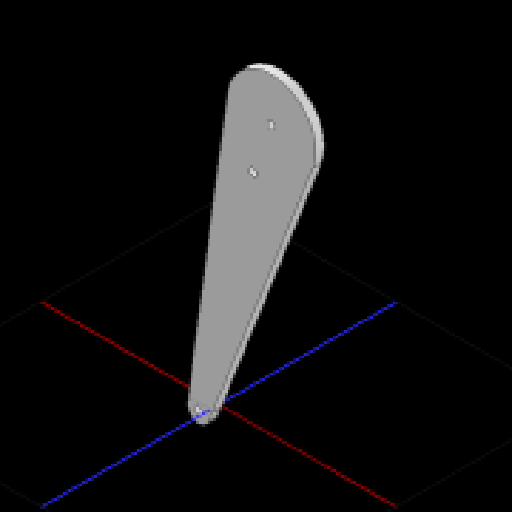
# Autodesk Inventor part: matchloaderbar
Saved by Autodesk Inventor 2025.2 (Build 292293000, 293)
## iProperties
Created: 2026-01-23
Part Number: matchloaderbar
Material: Generic
Document SubType Name: Modeling
Designer: cloudy
Density: 1 g/cm^3
Appearance: Default
Author: cloudy
Autodesk Inventor part; units mm, degrees
ref_plane "YZ Plane" through (0, 0, 0) normal (1, 0, 0) x (0, 1, 0)
ref_plane "XZ Plane" through (0, 0, 0) normal (0, 1, 0) x (-1, 0, 0)
ref_plane "XY Plane" through (0, 0, 0) normal (0, 0, 1) x (1, 0, 0)
sketch "Sketch1" plane through (0, 0, 0) normal (0, 0, 1) x (1, 0, 0)
  ellipse E0 centre (24.8761, 141.4019) end of major axis (27.0605, 141.4019) minor radius 2.1844 construction
  circle A0 centre (35.5142, 169.536) radius 3.175 construction
  circle A1 centre (-6.35, 7.62) radius 2.1209 construction
  arc A2 (59.2212, 160.418) -> (10.3749, 173.1659) centre (35.5142, 169.536) ccw
  arc A3 (-12.6593, 8.3379) -> (-0.4232, 5.3405) centre (-6.35, 7.62) ccw
  circle A4 centre (24.8761, 141.4019) radius 2.2479
  circle A5 centre (35.5142, 169.536) radius 2.2479
  circle A6 centre (-6.35, 7.62) radius 2.2479
  line L0 (-0.4232, 5.3405) -> (59.2212, 160.418)
  circle A7 centre (-5.0887, 32.7473) radius 2.2568
  arc A8 (-9.8023, 33.4279) -> (-5.7018, 37.4701) centre (-5.0887, 32.7473) ccw
  line L1 (-9.8206, 33.2857) -> (-12.6593, 8.3379)
  line L2 (-9.8023, 33.4279) -> (10.3749, 173.1659)
  point P0 (0, 0)
  dimension "d0" = 50.8
  dimension "d1" = 12.7
  dimension "d2" = 4.4958
  dimension "d3" = 4.4958
  dimension "d4" = 4.4958
  dimension "d7" = 4.5136
  dimension "d9" = 9.525
  constraints: 7 centre point, 7 point on circle, 6 coincident, 6 end point, 6 tangent
  measures "d0" diameter of A2
  measures "d1" diameter of A3
  measures "d2" diameter of A4
  measures "d3" diameter of A5
  measures "d4" diameter of A6
  measures "d7" diameter of A7
  measures "d9" diameter of A8
extrude "Extrusion1" add sketch "Sketch1" along normal blind 5.08
body "Solid1"
